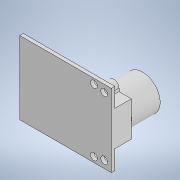
# Autodesk Inventor part: Техническое зрение OpenMV
Saved by Autodesk Inventor 2020 (Build 240168000, 168)
## iProperties
Created: 2019-06-16
Part Number: Техническое зрение OpenMV
Material: Типовые
Document SubType Name: Modeling
Designer: ШП
Density: 1 g/cm^3
Appearance: По умолчанию
Author: ШП
Autodesk Inventor part; units mm, degrees
ref_plane "YZ Plane" through (0, 0, 0) normal (1, 0, 0) x (0, 1, 0)
ref_plane "XZ Plane" through (0, 0, 0) normal (0, 1, 0) x (-1, 0, 0)
ref_plane "XY Plane" through (0, 0, 0) normal (0, 0, 1) x (1, 0, 0)
sketch "Эскиз1" plane through (0, 0, 0) normal (0, 0, 1) x (1, 0, 0)
  line L0 (0, 0) -> (44.5, 0)
  line L1 (44.5, 0) -> (44.5, 35.5)
  line L2 (44.5, 35.5) -> (0, 35.5)
  line L3 (0, 35.5) -> (0, 0)
  dimension "d0" = 44.5
  dimension "d1" = 35.5
  constraints: 8 end point, 2 parallel, 1 horizontal, 1 perpendicular
  measures "d0" distance of L2.end L1.end
  measures "d1" distance of L1.end L0.end
extrude "Выдавливание1" add sketch "Эскиз1" along normal blind 1.7
sketch "Эскиз2" plane through (0, 0, 1.7) normal (0, 0, 1) x (1, 0, 0)
  line L0 (0, 0) -> (44.5, 0) projected
  line L1 (44.5, 0) -> (44.5, 3.5)
  line L2 (44.5, 0) -> (44.5, 35.5) projected
  line L3 (44.5, 3.5) -> (41, 3.5)
  line L4 (44.5, 35.5) -> (44.5, 32)
  line L5 (44.5, 32) -> (41, 32)
  line L6 (44.5, 35.5) -> (0, 35.5) projected
  point P0 (36, 33)
  point P1 (36, 2.5)
  point P2 (36, 33)
  dimension "d4" = 3.5
  dimension "d5" = 3.5
  dimension "d6" = 3.5
  dimension "d7" = 3.5
  dimension "d26" = 8.5
  dimension "d27" = 8.5
  dimension "d28" = 2.5
  dimension "d29" = 2.5
  constraints: 8 end point, 2 perpendicular, 2 point on line, 1 coincident
  measures "d4" distance of L0.end L1.end
  measures "d5" distance of L1.end L3.end
  measures "d6" distance of L2.end L4.end
  measures "d7" distance of L4.end L5.end
  measures "d26" distance from line of L2 point (36, 33)
  measures "d27" distance from line of L2 point (36, 2.5)
  measures "d28" distance from line of L0 point (36, 2.5)
  measures "d29" distance from line of L6 point (36, 33)
hole "Отверстие1" at (41, 32, 1.7) at (41, 3.5, 1.7) at (36, 33, 1.7) at (36, 2.5, 1.7) direction (0, 0, -1) diameter 3.35 depth 15
sketch "Эскиз3" plane through (0, 0, 0) normal (0, 0, -1) x (-1, 0, 0)
  line L0 (-44.5, 0) -> (-44.5, 35.5) projected
  line L1 (-44.5, 0) -> (-44.5, 9.25)
  line L2 (-44.5, 9.25) -> (-27.5, 9.25)
  line L3 (-27.5, 9.25) -> (-27.5, 26.25)
  line L4 (-27.5, 26.25) -> (-44.5, 26.25)
  line L5 (-44.5, 26.25) -> (-44.5, 9.25)
  line L6 (-36, 26.25) -> (-36, 27.75)
  line L7 (-36, 9.25) -> (-36, 7.75)
  circle A0 centre (-36, 7.75) radius 2.5
  circle A1 centre (-36, 27.75) radius 2.5
  line L8 (-38.5, 27.75) -> (-33.5, 27.75)
  line L9 (-33.5, 27.75) -> (-33.5, 26.25)
  line L10 (-33.5, 26.25) -> (-38.5, 26.25)
  line L11 (-38.5, 26.25) -> (-38.5, 27.75)
  line L12 (-33.5, 7.75) -> (-38.5, 7.75)
  line L13 (-38.5, 7.75) -> (-38.5, 9.25)
  line L14 (-38.5, 9.25) -> (-33.5, 9.25)
  line L15 (-33.5, 9.25) -> (-33.5, 7.75)
  point P0 (0, 0)
  dimension "d20" = 5
  dimension "d21" = 5
  dimension "d15" = 9.25
  dimension "d16" = 17
  dimension "d17" = 17
  dimension "d18" = 1.5
  dimension "d19" = 1.5
  constraints: 30 end point, 6 parallel, 5 point on line, 3 horizontal, 3 perpendicular, 2 coincident, 2 midpoint, 2 vertical, 6 other
  measures "d15" distance of L0.start L1.end
  measures "d16" distance of L4.end L3.end
  measures "d17" distance of L3.end L2.end
  measures "d18" distance of L6.start L6.end
  measures "d19" distance of L7.start L7.end
extrude "Выдавливание2" add sketch "Эскиз3" along normal blind 8
sketch "Эскиз4" plane through (0, 0, -8) normal (0, 0, -1) x (-1, 0, 0)
  line L0 (-44.5, 0) -> (-44.5, 35.5) projected
  line L1 (-44.5, 17.75) -> (-27.5, 17.75)
  line L2 (-27.5, 26.25) -> (-27.5, 9.25) projected
  circle A0 centre (-36, 17.75) radius 8.5
  point P0 (0, 0)
  constraints: 3 midpoint, 2 end point, 1 horizontal alignment, 2 other
extrude "Выдавливание3" add sketch "Эскиз4" along normal blind 14
equation "\"d4\" = d6"
equation "\"d5\" = d6"
equation "\"d7\" = d6"
